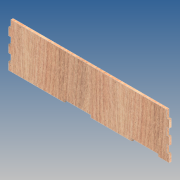
# Autodesk Inventor part: 2202_Housing Side_V1
Saved by Autodesk Inventor 2020 (Build 240168000, 168)
## iProperties
Created: 2019-11-08
Part Number: 2202_Housing Side_V1
Material: Wood (Birch)
Document SubType Name: Modeling
Designer: RFLab
Density: 0.55 g/cm^3
Appearance: Birch - Natural Polished
Author: RFLab
Autodesk Inventor part; units mm, degrees
ref_plane "YZ Plane" through (0, 0, 0) normal (1, 0, 0) x (0, 1, 0)
ref_plane "XZ Plane" through (0, 0, 0) normal (0, 1, 0) x (-1, 0, 0)
ref_plane "XY Plane" through (0, 0, 0) normal (0, 0, 1) x (1, 0, 0)
sketch "Sketch1" plane through (0, 0, 0) normal (0, 0, 1) x (1, 0, 0)
  line L0 (-215, 60) -> (215, 60)
  line L1 (215, 60) -> (215, -60)
  line L2 (215, -60) -> (-215, -60)
  line L3 (-215, -60) -> (-215, 60)
  point P0 (0, 0)
  dimension "d0" = 120
  dimension "d1" = 430
  dimension "d2" = 215
  dimension "d3" = 60
  constraints: 8 end point, 2 parallel, 1 horizontal, 1 perpendicular
  measures "d0" distance of L2.end L0.start
  measures "d1" distance of L0.start L0.end
  measures "d2" distance from line of L3 point (0, 0)
  measures "d3" distance from line of L2 point (0, 0)
extrude "Extrusion1" add sketch "Sketch1" along normal blind 6.35
sketch "Sketch2" plane through (0, 0, 6.35) normal (0, 0, 1) x (1, 0, 0)
  line L0 (215, 60) -> (-215, 60) projected
  line L1 (-215, 60) -> (-208.65, 60)
  line L2 (-208.65, 60) -> (-208.65, 40)
  line L3 (-208.65, 40) -> (-215, 40)
  line L4 (-215, 40) -> (-215, 60)
  line L5 (-215, 60) -> (-215, -60) projected
  line L6 (-215, 20) -> (-208.65, 20)
  line L7 (-208.65, 20) -> (-208.65, 0)
  line L8 (-208.65, 0) -> (-215, 0)
  line L9 (-215, 0) -> (-215, 20)
  line L10 (-215, -20) -> (-208.65, -20)
  line L11 (-208.65, -20) -> (-208.65, -40)
  line L12 (-208.65, -40) -> (-215, -40)
  line L13 (-215, -40) -> (-215, -20)
  line L14 (-215, -60) -> (-215, -55)
  line L15 (215, 60) -> (208.65, 60)
  line L16 (208.65, 60) -> (208.65, 40)
  line L17 (208.65, 40) -> (215, 40)
  line L18 (215, 40) -> (215, 60)
  line L19 (215, -60) -> (215, 60) projected
  line L20 (215, 20) -> (208.65, 20)
  line L21 (208.65, 20) -> (208.65, 0)
  line L22 (208.65, 0) -> (215, 0)
  line L23 (215, 0) -> (215, 20)
  line L24 (215, -20) -> (208.65, -20)
  line L25 (208.65, -20) -> (208.65, -40)
  line L26 (208.65, -40) -> (215, -40)
  line L27 (215, -40) -> (215, -20)
  line L28 (215, -60) -> (215, 60) projected
  line L29 (215, -60) -> (215, -55)
  point P0 (0, 0)
  point P1 (208.65, -60)
  dimension "d6" = 6.35
  dimension "d7" = 20
  dimension "d8" = 20
  dimension "d9" = 20
  dimension "d10" = 20
  dimension "d11" = 20
  dimension "d13" = 20
  dimension "d14" = 20
  dimension "d15" = 20
  dimension "d16" = 20
  dimension "d17" = 20
  dimension "d19" = 6.35
  constraints: 52 end point, 12 parallel, 11 point on line, 6 horizontal, 6 perpendicular
  measures "d6" distance of L0.end L1.end
  measures "d7" distance of L1.end L2.end
  measures "d8" distance of L6.end L2.end
  measures "d9" distance of L7.end L6.end
  measures "d10" distance of L10.end L7.end
  measures "d11" distance of L10.end L11.end
  measures "d13" distance of L15.end L16.end
  measures "d14" distance of L16.end L20.end
  measures "d15" distance of L20.end L21.end
  measures "d16" distance of L21.end L24.end
  measures "d17" distance of L24.end L25.end
  measures "d19" distance of L0.start L15.end
extrude "Extrusion2" cut sketch "Sketch2" against normal through all
sketch "Sketch3" plane through (0, 0, 6.35) normal (0, 0, 1) x (1, 0, 0)
  line L0 (-215, -60) -> (215, -60) projected
  line L1 (-65, -60) -> (5, -60)
  line L2 (5, -60) -> (5, -53.65)
  line L3 (5, -53.65) -> (-65, -53.65)
  line L4 (-65, -53.65) -> (-65, -60)
  line L5 (115, -60) -> (185, -60)
  line L6 (185, -60) -> (185, -53.65)
  line L7 (185, -53.65) -> (115, -53.65)
  line L8 (115, -53.65) -> (115, -60)
  point P0 (0, 0)
  point P1 (-268.65, -60)
  point P2 (268.65, -60)
  point P3 (185, -60)
  dimension "d22" = 70
  dimension "d23" = 70
  dimension "d25" = 110
  dimension "d26" = 6.35
  dimension "d27" = 6.35
  dimension "d30" = 150
  constraints: 16 end point, 4 parallel, 2 horizontal, 2 perpendicular, 2 point on line
  measures "d22" distance of L2.end L3.end
  measures "d23" distance of L6.end L7.end
  measures "d25" distance of L5.start L1.end
  measures "d26" distance of L5.end L6.end
  measures "d27" distance of L1.end L2.end
  measures "d30" distance of L0.start L1.start
extrude "Extrusion3" cut sketch "Sketch3" against normal through all
equation "\"d2\" = 0.5 * d1"
equation "\"d3\" = 0.5 * d0"
equation "\"d10\" = d8"
equation "\"d27\" = d26"
body "Solid1"
